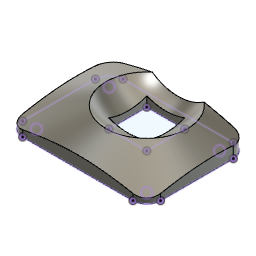
reset button guard v4 (Autodesk Fusion 360 design; units mm, degrees)
Autodesk Fusion 360 part; units mm, degrees
note: some values were not read from the file. Set by a fixed rule: which sketch regions a step uses.
sketch "top" plane through (0, 0, 0) normal (0, 1, 0) x (1, 0, 0)
  line L0 (2.75, -2.75) -> (-2.75, -2.75)
  line L1 (-2.75, -2.75) -> (-2.75, 2.75)
  line L2 (-2.75, 2.75) -> (2.75, 2.75)
  line L3 (2.75, 2.75) -> (2.75, -2.75)
  line L4 (2.75, -2.75) -> (-2.75, 2.75) construction
  line L5 (-2.75, -2.75) -> (2.75, 2.75) construction
  line L6 (-51.8482, 4.55) -> (53.2802, 4.55)
  line L7 (10, -10) -> (-10, -10)
  line L8 (-10, -10) -> (-10, 10)
  line L9 (-10, 10) -> (10, 10)
  line L10 (10, 10) -> (10, -10)
  line L11 (10, -10) -> (-10, 10) construction
  line L12 (-10, -10) -> (10, 10) construction
  line L13 (2.75, 2.75) -> (2.75, 4.55)
  line L14 (-2.75, 2.75) -> (-2.75, 4.55)
  dimension "d1" = 5.5
  dimension "d2" = 5.5
  dimension "d3" = 1.8
  dimension "d4" = 20
  dimension "d5" = 20
  constraint horizontal L0
  constraint perpendicular L0 L1
  constraint parallel L0 L2
  constraint parallel L1 L3
  constraint coincident L4 origin
  constraint coincident L5 origin
  constraint horizontal L6
  constraint horizontal L7
  constraint perpendicular L7 L8
  constraint parallel L7 L9
  constraint parallel L8 L10
  constraint coincident L11 origin
  constraint coincident L12 origin
  constraint coincident L6 L13.end
  constraint perpendicular L6 L13
  constraint coincident L6 L14.end
  constraint perpendicular L6 L14
  measures "d1" distance of L1.end L2.end
  measures "d2" distance of L0.end L1.end
  measures "d3" distance of L2 L6
  measures "d4" distance of L8.end L9.end
  measures "d5" distance of L7.end L8.end
extrude "Extrude1" add sketch "top" along normal blind 3 contours L0 L1 L3 L6 L7 L8 L10 L13 L14 | L2 L6 L13 L14
sketch "hole" plane through (0, 0, 0) normal (0, 0, 1) x (1, 0, 0)
  line L0 (0, 0) -> (0, 32.5783)
  circle A0 centre (0, 8.4) radius 8
  line L1 (0, 0.4) -> (15.5935, 0.4) construction
  line L2 (-10, 0) -> (10, 0) construction
  line L3 (10, 0) -> (10, 3) construction
  line L4 (10, 3) -> (-10, 3) construction
  line L5 (-10, 3) -> (-10, 0) construction
  line L6 (5.9025, 3) -> (10, 3)
  line L7 (5.9025, 3) -> (14.475, 0.4)
  line L8 (10, 3) -> (14.475, 3)
  line L9 (14.475, 3) -> (14.475, 0.4)
  point P0 (0, 0.4)
  point P1 (10, 0.4)
  dimension "d8" = 16
  dimension "d9" = 0.4
  constraint coincident L0.start origin
  constraint vertical L0
  constraint coincident L0 A0.centre
  constraint coincident A0 P0
  constraint coincident L0 P0
  constraint coincident P0 L1.start
  constraint tangent A0 L1
  constraint perpendicular L0 L1
  constraint coincident L1 P1
  constraint coincident L3 P1
  constraint coincident A0 L6.start
  constraint coincident L4 L6.start
  constraint coincident L3.end L4.start
  constraint coincident L1 L7.end
  constraint perpendicular L3 L8
  constraint perpendicular L1 L9
  measures "d8" diameter of A0
  measures "d9" distance of L0.start L1.start
revolve "Revolve1" cut sketch "hole" angle 360 about axis through (0, 0, 0) along (0, 1, 0) contours L6 L7 L8 L9 | L0 A0 picked at (2.6374, 8.0063)
fillet "Fillet1" radius 2 4 edges at (10, 0.2505, 10) (-10, 0.2505, 10) (-10, 0.729, -4.55) (10, 0.729, -4.55)
sketch "sticky" plane through (0, 0, 0) normal (0, 1, 0) x (1, 0, 0)
  arc A0 (10, 2.55) -> (8, 4.55) centre (8, 2.55) ccw
  line L0 (10, 2.55) -> (10, -8)
  arc A1 (8, -10) -> (10, -8) centre (8, -8) ccw
  line L1 (8, -10) -> (-8, -10)
  arc A2 (-10, -8) -> (-8, -10) centre (-8, -8) ccw
  line L2 (-10, -8) -> (-10, 2.55)
  arc A3 (-8, 4.55) -> (-10, 2.55) centre (-8, 2.55) ccw
  line L3 (-8, 4.55) -> (8, 4.55)
  line L4 (2.75, 2.75) -> (-2.75, 2.75)
  line L5 (-2.75, 2.75) -> (-2.75, -2.75)
  line L6 (-2.75, -2.75) -> (2.75, -2.75)
  line L7 (2.75, -2.75) -> (2.75, 2.75)
named bodies: "reset button guard"
